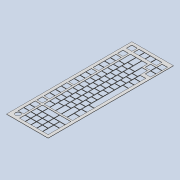
# Autodesk Inventor part: Layout
Saved by Autodesk Inventor 2021 (Build 250183000, 183)
## iProperties
Created: 2021-12-04
Part Number: Layout
Material: Generic
Document SubType Name: Modeling
Designer: Matthew Flooks
Density: 1 g/cm^3
Appearance: Default
Author: Matthew Flooks
Autodesk Inventor part; units mm, degrees
ref_plane "YZ Plane" through (0, 0, 0) normal (1, 0, 0) x (0, 1, 0)
ref_plane "XZ Plane" through (0, 0, 0) normal (0, 1, 0) x (-1, 0, 0)
ref_plane "XY Plane" through (0, 0, 0) normal (0, 0, 1) x (1, 0, 0)
sketch "Sketch1" plane through (0, 0, 0) normal (0, 1, 0) x (-1, 0, 0)
  line L0 (0, 0) -> (19, 0)
  line L1 (19, 0) -> (19, -39.05)
  line L2 (19, -39.05) -> (0, -39.05)
  line L3 (0, -39.05) -> (0, 0)
  line L4 (19, -40.1) -> (0, -40.1)
  line L5 (0, -40.1) -> (0, -59.1)
  line L6 (0, -59.1) -> (19, -59.1)
  line L7 (19, -59.1) -> (19, -40.1)
  line L8 (0, -60.15) -> (39.05, -60.15)
  line L9 (39.05, -60.15) -> (39.05, -79.15)
  line L10 (39.05, -79.15) -> (0, -79.15)
  line L11 (0, -79.15) -> (0, -60.15)
  line L12 (20.05, -59.1) -> (39.05, -59.1)
  line L13 (39.05, -59.1) -> (39.05, -40.1)
  line L14 (39.05, -40.1) -> (20.05, -40.1)
  line L15 (20.05, -40.1) -> (20.05, -59.1)
  line L16 (20.05, -39.05) -> (39.05, -39.05)
  line L17 (39.05, -39.05) -> (39.05, -20.05)
  line L18 (39.05, -20.05) -> (20.05, -20.05)
  line L19 (20.05, -20.05) -> (20.05, -39.05)
  line L20 (20.05, -19) -> (39.05, -19)
  line L21 (39.05, -19) -> (39.05, 0)
  line L22 (39.05, 0) -> (20.05, 0)
  line L23 (20.05, 0) -> (20.05, -19)
  line L24 (40.1, 0) -> (59.1, 0)
  line L25 (59.1, 0) -> (59.1, -19)
  line L26 (59.1, -19) -> (40.1, -19)
  line L27 (40.1, -19) -> (40.1, 0)
  line L28 (40.1, -20.05) -> (59.1, -20.05)
  line L29 (59.1, -20.05) -> (59.1, -39.05)
  line L30 (59.1, -39.05) -> (40.1, -39.05)
  line L31 (40.1, -39.05) -> (40.1, -20.05)
  line L32 (40.1, -40.1) -> (59.1, -40.1)
  line L33 (59.1, -40.1) -> (59.1, -59.1)
  line L34 (59.1, -59.1) -> (40.1, -59.1)
  line L35 (40.1, -59.1) -> (40.1, -40.1)
  line L36 (40.1, -60.15) -> (79.15, -60.15)
  line L37 (79.15, -60.15) -> (79.15, -79.15)
  line L38 (79.15, -79.15) -> (40.1, -79.15)
  line L39 (40.1, -79.15) -> (40.1, -60.15)
  line L40 (60.15, -59.1) -> (79.15, -59.1)
  line L41 (79.15, -59.1) -> (79.15, -40.1)
  line L42 (79.15, -40.1) -> (60.15, -40.1)
  line L43 (60.15, -40.1) -> (60.15, -59.1)
  line L44 (60.15, -39.05) -> (79.15, -39.05)
  line L45 (79.15, -39.05) -> (79.15, -20.05)
  line L46 (79.15, -20.05) -> (60.15, -20.05)
  line L47 (60.15, -20.05) -> (60.15, -39.05)
  line L48 (60.15, -19) -> (79.15, -19)
  line L49 (79.15, -19) -> (79.15, 0)
  line L50 (79.15, 0) -> (60.15, 0)
  line L51 (60.15, 0) -> (60.15, -19)
  line L52 (80.2, 0) -> (99.2, 0)
  line L53 (99.2, 0) -> (99.2, -19)
  line L54 (99.2, -19) -> (80.2, -19)
  line L55 (80.2, -19) -> (80.2, 0)
  line L56 (80.2, -20.05) -> (99.2, -20.05)
  line L57 (99.2, -20.05) -> (99.2, -39.05)
  line L58 (99.2, -39.05) -> (80.2, -39.05)
  line L59 (80.2, -39.05) -> (80.2, -20.05)
  line L60 (80.2, -40.1) -> (99.2, -40.1)
  line L61 (99.2, -40.1) -> (99.2, -59.1)
  line L62 (99.2, -59.1) -> (80.2, -59.1)
  line L63 (80.2, -59.1) -> (80.2, -40.1)
  line L64 (80.2, -60.15) -> (99.2, -60.15)
  line L65 (99.2, -60.15) -> (99.2, -79.15)
  line L66 (99.2, -79.15) -> (80.2, -79.15)
  line L67 (80.2, -79.15) -> (80.2, -60.15)
  line L68 (105.0125, -20.05) -> (124.0125, -20.05)
  line L69 (124.0125, -20.05) -> (124.0125, -39.05)
  line L70 (124.0125, -39.05) -> (105.0125, -39.05)
  line L71 (105.0125, -39.05) -> (105.0125, -20.05)
  line L72 (105.0125, -40.1) -> (124.0125, -40.1)
  line L73 (124.0125, -40.1) -> (124.0125, -59.1)
  line L74 (124.0125, -59.1) -> (105.0125, -59.1)
  line L75 (105.0125, -59.1) -> (105.0125, -40.1)
  line L76 (105.0125, -60.15) -> (124.0125, -60.15)
  line L77 (124.0125, -60.15) -> (124.0125, -79.15)
  line L78 (124.0125, -79.15) -> (105.0125, -79.15)
  line L79 (105.0125, -79.15) -> (105.0125, -60.15)
  line L80 (0, -84.9625) -> (19, -84.9625)
  line L81 (19, -84.9625) -> (19, -108.975)
  line L82 (19, -108.975) -> (0, -108.975)
  line L83 (0, -108.975) -> (0, -84.9625)
  line L84 (0, -110.025) -> (19, -110.025)
  line L85 (19, -110.025) -> (19, -134.0375)
  line L86 (19, -134.0375) -> (0, -134.0375)
  line L87 (0, -134.0375) -> (0, -110.025)
  line L88 (0, -135.0875) -> (19, -135.0875)
  line L89 (19, -135.0875) -> (19, -159.1)
  line L90 (19, -159.1) -> (0, -159.1)
  line L91 (0, -159.1) -> (0, -135.0875)
  line L92 (0, -160.15) -> (19, -160.15)
  line L93 (19, -160.15) -> (19, -278.15)
  line L94 (19, -278.15) -> (0, -278.15)
  line L95 (0, -278.15) -> (0, -160.15)
  line L96 (0, -279.2) -> (19, -279.2)
  line L97 (19, -279.2) -> (19, -298.2)
  line L98 (19, -298.2) -> (0, -298.2)
  line L99 (0, -298.2) -> (0, -279.2)
  line L100 (0, -299.25) -> (19, -299.25)
  line L101 (19, -299.25) -> (19, -318.25)
  line L102 (19, -318.25) -> (0, -318.25)
  line L103 (0, -318.25) -> (0, -299.25)
  line L104 (0, -319.3) -> (19, -319.3)
  line L105 (19, -319.3) -> (19, -338.3)
  line L106 (19, -338.3) -> (0, -338.3)
  line L107 (0, -338.3) -> (0, -319.3)
  line L108 (20.05, -84.9625) -> (39.05, -84.9625)
  line L109 (39.05, -84.9625) -> (39.05, -129.025)
  line L110 (39.05, -129.025) -> (20.05, -129.025)
  line L111 (20.05, -129.025) -> (20.05, -84.9625)
  line L112 (40.1, -84.9625) -> (59.1, -84.9625)
  line L113 (59.1, -84.9625) -> (59.1, -119)
  line L114 (59.1, -119) -> (40.1, -119)
  line L115 (40.1, -119) -> (40.1, -84.9625)
  line L116 (60.15, -84.9625) -> (79.15, -84.9625)
  line L117 (79.15, -84.9625) -> (79.15, -113.9875)
  line L118 (79.15, -113.9875) -> (60.15, -113.9875)
  line L119 (60.15, -113.9875) -> (60.15, -84.9625)
  line L120 (80.2, -84.9625) -> (99.2, -84.9625)
  line L121 (99.2, -84.9625) -> (99.2, -103.9625)
  line L122 (99.2, -103.9625) -> (80.2, -103.9625)
  line L123 (80.2, -103.9625) -> (80.2, -84.9625)
  line L124 (20.05, -130.075) -> (39.05, -130.075)
  line L125 (39.05, -130.075) -> (39.05, -149.075)
  line L126 (39.05, -149.075) -> (20.05, -149.075)
  line L127 (20.05, -149.075) -> (20.05, -130.075)
  line L128 (20.05, -150.125) -> (39.05, -150.125)
  line L129 (39.05, -150.125) -> (39.05, -169.125)
  line L130 (39.05, -169.125) -> (20.05, -169.125)
  line L131 (20.05, -169.125) -> (20.05, -150.125)
  line L132 (20.05, -170.175) -> (39.05, -170.175)
  line L133 (39.05, -170.175) -> (39.05, -189.175)
  line L134 (39.05, -189.175) -> (20.05, -189.175)
  line L135 (20.05, -189.175) -> (20.05, -170.175)
  line L136 (20.05, -190.225) -> (39.05, -190.225)
  line L137 (39.05, -190.225) -> (39.05, -209.225)
  line L138 (39.05, -209.225) -> (20.05, -209.225)
  line L139 (20.05, -209.225) -> (20.05, -190.225)
  line L140 (20.05, -210.275) -> (39.05, -210.275)
  line L141 (39.05, -210.275) -> (39.05, -229.275)
  line L142 (39.05, -229.275) -> (20.05, -229.275)
  line L143 (20.05, -229.275) -> (20.05, -210.275)
  line L144 (20.05, -230.325) -> (39.05, -230.325)
  line L145 (39.05, -230.325) -> (39.05, -249.325)
  line L146 (39.05, -249.325) -> (20.05, -249.325)
  line L147 (20.05, -249.325) -> (20.05, -230.325)
  line L148 (20.05, -250.375) -> (39.05, -250.375)
  line L149 (39.05, -250.375) -> (39.05, -269.375)
  line L150 (39.05, -269.375) -> (20.05, -269.375)
  line L151 (20.05, -269.375) -> (20.05, -250.375)
  line L152 (20.05, -270.425) -> (39.05, -270.425)
  line L153 (39.05, -270.425) -> (39.05, -289.425)
  line L154 (39.05, -289.425) -> (20.05, -289.425)
  line L155 (20.05, -289.425) -> (20.05, -270.425)
  line L156 (20.05, -290.475) -> (39.05, -290.475)
  line L157 (39.05, -290.475) -> (39.05, -309.475)
  line L158 (39.05, -309.475) -> (20.05, -309.475)
  line L159 (20.05, -309.475) -> (20.05, -290.475)
  line L160 (20.05, -329.525) -> (39.05, -329.525)
  line L161 (39.05, -329.525) -> (39.05, -310.525)
  line L162 (39.05, -310.525) -> (20.05, -310.525)
  line L163 (20.05, -310.525) -> (20.05, -329.525)
  line L164 (20.05, -330.575) -> (39.05, -330.575)
  line L165 (39.05, -330.575) -> (39.05, -364.6125)
  line L166 (39.05, -364.6125) -> (20.05, -364.6125)
  line L167 (20.05, -364.6125) -> (20.05, -330.575)
  line L168 (40.1, -120.05) -> (59.1, -120.05)
  line L169 (59.1, -120.05) -> (59.1, -139.05)
  line L170 (59.1, -139.05) -> (40.1, -139.05)
  line L171 (40.1, -139.05) -> (40.1, -120.05)
  line L172 (40.1, -140.1) -> (59.1, -140.1)
  line L173 (59.1, -140.1) -> (59.1, -159.1)
  line L174 (59.1, -159.1) -> (40.1, -159.1)
  line L175 (40.1, -159.1) -> (40.1, -140.1)
  line L176 (40.1, -160.15) -> (59.1, -160.15)
  line L177 (59.1, -160.15) -> (59.1, -179.15)
  line L178 (59.1, -179.15) -> (40.1, -179.15)
  line L179 (40.1, -179.15) -> (40.1, -160.15)
  line L180 (40.1, -180.2) -> (59.1, -180.2)
  line L181 (59.1, -180.2) -> (59.1, -199.2)
  line L182 (59.1, -199.2) -> (40.1, -199.2)
  line L183 (40.1, -199.2) -> (40.1, -180.2)
  line L184 (40.1, -200.25) -> (59.1, -200.25)
  line L185 (59.1, -200.25) -> (59.1, -219.25)
  line L186 (59.1, -219.25) -> (40.1, -219.25)
  line L187 (40.1, -219.25) -> (40.1, -200.25)
  line L188 (59.1, -220.3) -> (40.1, -220.3)
  line L189 (40.1, -220.3) -> (40.1, -239.3)
  line L190 (40.1, -239.3) -> (59.1, -239.3)
  line L191 (59.1, -239.3) -> (59.1, -220.3)
  line L192 (40.1, -240.35) -> (59.1, -240.35)
  line L193 (59.1, -240.35) -> (59.1, -259.35)
  line L194 (59.1, -259.35) -> (40.1, -259.35)
  line L195 (40.1, -259.35) -> (40.1, -240.35)
  line L196 (40.1, -260.4) -> (59.1, -260.4)
  line L197 (59.1, -260.4) -> (59.1, -279.4)
  line L198 (59.1, -279.4) -> (40.1, -279.4)
  line L199 (40.1, -279.4) -> (40.1, -260.4)
  line L200 (40.1, -280.45) -> (59.1, -280.45)
  line L201 (59.1, -280.45) -> (59.1, -299.45)
  line L202 (59.1, -299.45) -> (40.1, -299.45)
  line L203 (40.1, -299.45) -> (40.1, -280.45)
  line L204 (40.1, -300.5) -> (59.1, -300.5)
  line L205 (59.1, -300.5) -> (59.1, -319.5)
  line L206 (59.1, -319.5) -> (40.1, -319.5)
  line L207 (40.1, -319.5) -> (40.1, -300.5)
  line L208 (40.1, -320.55) -> (59.1, -320.55)
  line L209 (59.1, -320.55) -> (59.1, -339.55)
  line L210 (59.1, -339.55) -> (40.1, -339.55)
  line L211 (40.1, -339.55) -> (40.1, -320.55)
  line L212 (40.1, -340.6) -> (59.1, -340.6)
  line L213 (59.1, -340.6) -> (59.1, -384.6625)
  line L214 (59.1, -384.6625) -> (40.1, -384.6625)
  line L215 (40.1, -384.6625) -> (40.1, -340.6)
  line L216 (79.15, -115.0375) -> (60.15, -115.0375)
  line L217 (60.15, -115.0375) -> (60.15, -134.0375)
  line L218 (60.15, -134.0375) -> (79.15, -134.0375)
  line L219 (79.15, -134.0375) -> (79.15, -115.0375)
  line L220 (79.15, -135.0875) -> (60.15, -135.0875)
  line L221 (60.15, -135.0875) -> (60.15, -154.0875)
  line L222 (60.15, -154.0875) -> (79.15, -154.0875)
  line L223 (79.15, -154.0875) -> (79.15, -135.0875)
  line L224 (79.15, -155.1375) -> (60.15, -155.1375)
  line L225 (60.15, -155.1375) -> (60.15, -174.1375)
  line L226 (60.15, -174.1375) -> (79.15, -174.1375)
  line L227 (79.15, -174.1375) -> (79.15, -155.1375)
  line L228 (79.15, -175.1875) -> (60.15, -175.1875)
  line L229 (60.15, -175.1875) -> (60.15, -194.1875)
  line L230 (60.15, -194.1875) -> (79.15, -194.1875)
  line L231 (79.15, -194.1875) -> (79.15, -175.1875)
  line L232 (79.15, -195.2375) -> (60.15, -195.2375)
  line L233 (60.15, -195.2375) -> (60.15, -214.2375)
  line L234 (60.15, -214.2375) -> (79.15, -214.2375)
  line L235 (79.15, -214.2375) -> (79.15, -195.2375)
  line L236 (79.15, -215.2875) -> (60.15, -215.2875)
  line L237 (60.15, -215.2875) -> (60.15, -234.2875)
  line L238 (60.15, -234.2875) -> (79.15, -234.2875)
  line L239 (79.15, -234.2875) -> (79.15, -215.2875)
  line L240 (79.15, -235.3375) -> (60.15, -235.3375)
  line L241 (60.15, -235.3375) -> (60.15, -254.3375)
  line L242 (60.15, -254.3375) -> (79.15, -254.3375)
  line L243 (79.15, -254.3375) -> (79.15, -235.3375)
  line L244 (79.15, -255.3875) -> (60.15, -255.3875)
  line L245 (60.15, -255.3875) -> (60.15, -274.3875)
  line L246 (60.15, -274.3875) -> (79.15, -274.3875)
  line L247 (79.15, -274.3875) -> (79.15, -255.3875)
  line L248 (79.15, -275.4375) -> (60.15, -275.4375)
  line L249 (60.15, -275.4375) -> (60.15, -294.4375)
  line L250 (60.15, -294.4375) -> (79.15, -294.4375)
  line L251 (79.15, -294.4375) -> (79.15, -275.4375)
  line L252 (79.15, -295.4875) -> (60.15, -295.4875)
  line L253 (60.15, -295.4875) -> (60.15, -314.4875)
  line L254 (60.15, -314.4875) -> (79.15, -314.4875)
  line L255 (79.15, -314.4875) -> (79.15, -295.4875)
  line L256 (60.15, -315.5375) -> (79.15, -315.5375)
  line L257 (79.15, -315.5375) -> (79.15, -334.5375)
  line L258 (79.15, -334.5375) -> (60.15, -334.5375)
  line L259 (60.15, -334.5375) -> (60.15, -315.5375)
  line L260 (60.15, -335.5875) -> (79.15, -335.5875)
  line L261 (79.15, -335.5875) -> (79.15, -354.5875)
  line L262 (79.15, -354.5875) -> (60.15, -354.5875)
  line L263 (60.15, -354.5875) -> (60.15, -335.5875)
  line L264 (79.15, -355.6375) -> (60.15, -355.6375)
  line L265 (60.15, -355.6375) -> (60.15, -384.6625)
  line L266 (60.15, -384.6625) -> (79.15, -384.6625)
  line L267 (79.15, -384.6625) -> (79.15, -355.6375)
  line L268 (80.2, -105.0125) -> (99.2, -105.0125)
  line L269 (99.2, -105.0125) -> (99.2, -124.0125)
  line L270 (99.2, -124.0125) -> (80.2, -124.0125)
  line L271 (80.2, -124.0125) -> (80.2, -105.0125)
  line L272 (80.2, -125.0625) -> (99.2, -125.0625)
  line L273 (99.2, -125.0625) -> (99.2, -144.0625)
  line L274 (99.2, -144.0625) -> (80.2, -144.0625)
  line L275 (80.2, -144.0625) -> (80.2, -125.0625)
  line L276 (80.2, -145.1125) -> (99.2, -145.1125)
  line L277 (99.2, -145.1125) -> (99.2, -164.1125)
  line L278 (99.2, -164.1125) -> (80.2, -164.1125)
  line L279 (80.2, -164.1125) -> (80.2, -145.1125)
  line L280 (80.2, -165.1625) -> (99.2, -165.1625)
  line L281 (99.2, -165.1625) -> (99.2, -184.1625)
  line L282 (99.2, -184.1625) -> (80.2, -184.1625)
  line L283 (80.2, -184.1625) -> (80.2, -165.1625)
  line L284 (80.2, -185.2125) -> (99.2, -185.2125)
  line L285 (99.2, -185.2125) -> (99.2, -204.2125)
  line L286 (99.2, -204.2125) -> (80.2, -204.2125)
  line L287 (80.2, -204.2125) -> (80.2, -185.2125)
  line L288 (80.2, -205.2625) -> (99.2, -205.2625)
  line L289 (99.2, -205.2625) -> (99.2, -224.2625)
  line L290 (99.2, -224.2625) -> (80.2, -224.2625)
  line L291 (80.2, -224.2625) -> (80.2, -205.2625)
  line L292 (80.2, -225.3125) -> (99.2, -225.3125)
  line L293 (99.2, -225.3125) -> (99.2, -244.3125)
  line L294 (99.2, -244.3125) -> (80.2, -244.3125)
  line L295 (80.2, -244.3125) -> (80.2, -225.3125)
  line L296 (80.2, -245.3625) -> (99.2, -245.3625)
  line L297 (99.2, -245.3625) -> (99.2, -264.3625)
  line L298 (99.2, -264.3625) -> (80.2, -264.3625)
  line L299 (80.2, -264.3625) -> (80.2, -245.3625)
  line L300 (80.2, -265.4125) -> (99.2, -265.4125)
  line L301 (99.2, -265.4125) -> (99.2, -284.4125)
  line L302 (99.2, -284.4125) -> (80.2, -284.4125)
  line L303 (80.2, -284.4125) -> (80.2, -265.4125)
  line L304 (80.2, -285.4625) -> (99.2, -285.4625)
  line L305 (99.2, -285.4625) -> (99.2, -304.4625)
  line L306 (99.2, -304.4625) -> (80.2, -304.4625)
  line L307 (80.2, -304.4625) -> (80.2, -285.4625)
  line L308 (80.2, -305.5125) -> (99.2, -305.5125)
  line L309 (99.2, -305.5125) -> (99.2, -324.5125)
  line L310 (99.2, -324.5125) -> (80.2, -324.5125)
  line L311 (80.2, -324.5125) -> (80.2, -305.5125)
  line L312 (80.2, -325.5625) -> (99.2, -325.5625)
  line L313 (99.2, -325.5625) -> (99.2, -344.5625)
  line L314 (99.2, -344.5625) -> (80.2, -344.5625)
  line L315 (80.2, -344.5625) -> (80.2, -325.5625)
  line L316 (80.2, -345.6125) -> (99.2, -345.6125)
  line L317 (99.2, -345.6125) -> (99.2, -384.6625)
  line L318 (99.2, -384.6625) -> (80.2, -384.6625)
  line L319 (80.2, -384.6625) -> (80.2, -345.6125)
  line L320 (105.0125, -84.9625) -> (124.0125, -84.9625)
  line L321 (124.0125, -84.9625) -> (124.0125, -103.9625)
  line L322 (124.0125, -103.9625) -> (105.0125, -103.9625)
  line L323 (105.0125, -103.9625) -> (105.0125, -84.9625)
  line L324 (124.0125, -109.775) -> (105.0125, -109.775)
  line L325 (105.0125, -109.775) -> (105.0125, -128.775)
  line L326 (105.0125, -128.775) -> (124.0125, -128.775)
  line L327 (124.0125, -128.775) -> (124.0125, -109.775)
  line L328 (124.0125, -129.825) -> (105.0125, -129.825)
  line L329 (105.0125, -129.825) -> (105.0125, -148.825)
  line L330 (105.0125, -148.825) -> (124.0125, -148.825)
  line L331 (124.0125, -148.825) -> (124.0125, -129.825)
  line L332 (124.0125, -149.875) -> (105.0125, -149.875)
  line L333 (105.0125, -149.875) -> (105.0125, -168.875)
  line L334 (105.0125, -168.875) -> (124.0125, -168.875)
  line L335 (124.0125, -168.875) -> (124.0125, -149.875)
  line L336 (124.0125, -169.925) -> (105.0125, -169.925)
  line L337 (105.0125, -169.925) -> (105.0125, -188.925)
  line L338 (105.0125, -188.925) -> (124.0125, -188.925)
  line L339 (124.0125, -188.925) -> (124.0125, -169.925)
  line L340 (124.0125, -213.7375) -> (105.0125, -213.7375)
  line L341 (105.0125, -213.7375) -> (105.0125, -194.7375)
  line L342 (105.0125, -194.7375) -> (124.0125, -194.7375)
  line L343 (124.0125, -194.7375) -> (124.0125, -213.7375)
  line L344 (124.0125, -214.7875) -> (105.0125, -214.7875)
  line L345 (105.0125, -214.7875) -> (105.0125, -233.7875)
  line L346 (105.0125, -233.7875) -> (124.0125, -233.7875)
  line L347 (124.0125, -233.7875) -> (124.0125, -214.7875)
  line L348 (124.0125, -234.8375) -> (105.0125, -234.8375)
  line L349 (105.0125, -234.8375) -> (105.0125, -253.8375)
  line L350 (105.0125, -253.8375) -> (124.0125, -253.8375)
  line L351 (124.0125, -253.8375) -> (124.0125, -234.8375)
  line L352 (124.0125, -254.8875) -> (105.0125, -254.8875)
  line L353 (105.0125, -254.8875) -> (105.0125, -273.8875)
  line L354 (105.0125, -273.8875) -> (124.0125, -273.8875)
  line L355 (124.0125, -273.8875) -> (124.0125, -254.8875)
  line L356 (124.0125, -279.7) -> (105.0125, -279.7)
  line L357 (105.0125, -279.7) -> (105.0125, -298.7)
  line L358 (105.0125, -298.7) -> (124.0125, -298.7)
  line L359 (124.0125, -298.7) -> (124.0125, -279.7)
  line L360 (124.0125, -299.75) -> (105.0125, -299.75)
  line L361 (105.0125, -299.75) -> (105.0125, -318.75)
  line L362 (105.0125, -318.75) -> (124.0125, -318.75)
  line L363 (124.0125, -318.75) -> (124.0125, -299.75)
  line L364 (124.0125, -319.8) -> (105.0125, -319.8)
  line L365 (105.0125, -319.8) -> (105.0125, -338.8)
  line L366 (105.0125, -338.8) -> (124.0125, -338.8)
  line L367 (124.0125, -338.8) -> (124.0125, -319.8)
  line L368 (124.0125, -339.85) -> (105.0125, -339.85)
  line L369 (105.0125, -339.85) -> (105.0125, -358.85)
  line L370 (105.0125, -358.85) -> (124.0125, -358.85)
  line L371 (124.0125, -358.85) -> (124.0125, -339.85)
  line L372 (124.0125, -364.6625) -> (105.0125, -364.6625)
  line L373 (105.0125, -364.6625) -> (105.0125, -383.6625)
  line L374 (105.0125, -383.6625) -> (124.0125, -383.6625)
  line L375 (124.0125, -383.6625) -> (124.0125, -364.6625)
  line L376 (124.0125, -395.2375) -> (105.0125, -395.2375)
  line L377 (105.0125, -395.2375) -> (105.0125, -414.2375)
  line L378 (105.0125, -414.2375) -> (124.0125, -414.2375)
  line L379 (124.0125, -414.2375) -> (124.0125, -395.2375)
  line L380 (14.2375, -350.375) -> (-4.7625, -350.375)
  line L381 (-4.7625, -350.375) -> (-4.7625, -369.375)
  line L382 (-4.7625, -369.375) -> (14.2375, -369.375)
  line L383 (14.2375, -369.375) -> (14.2375, -350.375)
  line L384 (14.2375, -370.425) -> (-4.7625, -370.425)
  line L385 (-4.7625, -370.425) -> (-4.7625, -389.425)
  line L386 (-4.7625, -389.425) -> (14.2375, -389.425)
  line L387 (14.2375, -389.425) -> (14.2375, -370.425)
  line L388 (14.2375, -390.475) -> (-4.7625, -390.475)
  line L389 (-4.7625, -390.475) -> (-4.7625, -409.475)
  line L390 (-4.7625, -409.475) -> (14.2375, -409.475)
  line L391 (14.2375, -409.475) -> (14.2375, -390.475)
  line L392 (15.2875, -389.425) -> (34.2875, -389.425)
  line L393 (34.2875, -389.425) -> (34.2875, -370.425)
  line L394 (34.2875, -370.425) -> (15.2875, -370.425)
  line L395 (15.2875, -370.425) -> (15.2875, -389.425)
  line L396 (20.05, -395.2375) -> (39.05, -395.2375)
  line L397 (39.05, -395.2375) -> (39.05, -414.2375)
  line L398 (39.05, -414.2375) -> (20.05, -414.2375)
  line L399 (20.05, -414.2375) -> (20.05, -395.2375)
  line L400 (60.15, -395.2375) -> (79.15, -395.2375)
  line L401 (79.15, -395.2375) -> (79.15, -414.2375)
  line L402 (79.15, -414.2375) -> (60.15, -414.2375)
  line L403 (60.15, -414.2375) -> (60.15, -395.2375)
  line L404 (80.2, -395.2375) -> (99.2, -395.2375)
  line L405 (99.2, -395.2375) -> (99.2, -414.2375)
  line L406 (99.2, -414.2375) -> (80.2, -414.2375)
  line L407 (80.2, -414.2375) -> (80.2, -395.2375)
  line L408 (59.1, -395.2375) -> (40.1, -395.2375)
  line L409 (40.1, -395.2375) -> (40.1, -414.2375)
  line L410 (40.1, -414.2375) -> (59.1, -414.2375)
  line L411 (59.1, -414.2375) -> (59.1, -395.2375)
  circle A0 centre (114.5125, -10) radius 8.525
  line L412 (-10, 10) -> (134.0125, 10)
  line L413 (134.0125, 10) -> (134.0125, -424.2375)
  line L414 (134.0125, -424.2375) -> (-10, -424.2375)
  line L415 (-10, -424.2375) -> (-10, 10)
  line L416 (114.5125, -20.05) -> (114.5125, -10) construction
  point P0 (0, 0)
  dimension "d0" = 39.05
  dimension "d1" = 19
  dimension "d2" = 0
  dimension "d3" = 0
  dimension "d4" = 19
  dimension "d5" = 1.05
  dimension "d6" = 39.05
  dimension "d7" = 19
  dimension "d8" = 1.05
  dimension "d10" = 19
  dimension "d12" = 19
  dimension "d13" = 19
  dimension "d15" = 19
  dimension "d16" = 19
  dimension "d17" = 1.05
  dimension "d18" = 1.05
  dimension "d21" = 19
  dimension "d25" = 1.05
  dimension "d26" = 39.05
  dimension "d27" = 19
  dimension "d33" = 1.05
  dimension "d34" = 19
  dimension "d37" = 24.0125
  dimension "d38" = 5.8125
  dimension "d39" = 24.0125
  dimension "d40" = 24.0125
  dimension "d41" = 1.05
  dimension "d42" = 1.05
  dimension "d43" = 1.05
  dimension "d44" = 1.05
  dimension "d45" = 1.05
  dimension "d46" = 1.05
  dimension "d47" = 19
  dimension "d48" = 19
  dimension "d49" = 19
  dimension "d50" = 118
  dimension "d51" = 44.0625
  dimension "d52" = 1.05
  dimension "d53" = 34.0375
  dimension "d54" = 29.025
  dimension "d55" = 19
  dimension "d56" = 1.05
  dimension "d57" = 1.05
  dimension "d58" = 1.05
  dimension "d59" = 1.05
  dimension "d60" = 1.05
  dimension "d61" = 1.05
  dimension "d62" = 1.05
  dimension "d63" = 1.05
  dimension "d64" = 1.05
  dimension "d66" = 19
  dimension "d67" = 19
  dimension "d68" = 19
  dimension "d69" = 19
  dimension "d70" = 19
  dimension "d71" = 19
  dimension "d72" = 19
  dimension "d73" = 19
  dimension "d74" = 19
  dimension "d75" = 19
  dimension "d76" = 1.05
  dimension "d77" = 1.05
  dimension "d78" = 34.0375
  dimension "d79" = 19
  constraints: 834 end point, 208 parallel, 139 point on line, 104 horizontal, 104 perpendicular, 76 collinear, 1 centre point, 1 midpoint, 1 vertical
  measures "d0" distance of L2.end L0.start
  measures "d1" distance of L1.end L2.end
  measures "d2" distance from line of point (0, 0) L0
  measures "d3" distance from line of point (0, 0) L3
  measures "d4" distance of L4.end L5.end
  measures "d5" distance between parallel lines of L2 L4
  measures "d6" distance of L9.end L10.end
  measures "d7" distance of L10.end L8.start
  measures "d8" distance between parallel lines of L6 L8
  measures "d10" distance of L12.end L13.end
  measures "d12" distance of L17.end L18.end
  measures "d13" distance of L16.end L17.end
  measures "d15" distance of L20.end L21.end
  measures "d16" distance of L21.end L22.end
  measures "d17" distance between parallel lines of L1 L23
  measures "d18" distance between parallel lines of L18 L20
  measures "d21" distance of L24.start L24.end
  measures "d25" distance between parallel lines of L21 L27
  measures "d26" distance of L37.end L38.end
  measures "d27" distance of L41.end L42.end
  measures "d33" distance between parallel lines of L41 L63
  measures "d34" distance of L52.start L52.end
  measures "d37" distance of L82.end L80.start
  measures "d38" distance between parallel lines of L10 L80
  measures "d39" distance of L86.end L84.start
  measures "d40" distance of L90.end L88.start
  measures "d41" distance between parallel lines of L82 L84
  measures "d42" distance between parallel lines of L88 L86
  measures "d43" distance between parallel lines of L92 L90
  measures "d44" distance between parallel lines of L96 L94
  measures "d45" distance between parallel lines of L100 L98
  measures "d46" distance between parallel lines of L104 L102
  measures "d47" distance of L98.end L96.start
  measures "d48" distance of L102.end L100.start
  measures "d49" distance of L106.end L104.start
  measures "d50" distance of L94.end L92.start
  measures "d51" distance of L110.end L108.start
  measures "d52" distance between parallel lines of L111 L81
  measures "d53" distance of L114.end L112.start
  measures "d54" distance of L118.end L116.start
  measures "d55" distance of L122.end L120.start
  measures "d56" distance between parallel lines of L124 L110
  measures "d57" distance between parallel lines of L128 L126
  measures "d58" distance between parallel lines of L132 L130
  measures "d59" distance between parallel lines of L136 L134
  measures "d60" distance between parallel lines of L140 L138
  measures "d61" distance between parallel lines of L144 L142
  measures "d62" distance between parallel lines of L148 L146
  measures "d63" distance between parallel lines of L152 L150
  measures "d64" distance between parallel lines of L156 L154
  measures "d66" distance of L126.end L124.start
  measures "d67" distance of L130.end L128.start
  measures "d68" distance of L134.end L132.start
  measures "d69" distance of L138.end L136.start
  measures "d70" distance of L142.end L140.start
  measures "d71" distance of L146.end L144.start
  measures "d72" distance of L150.end L148.start
  measures "d73" distance of L154.end L152.start
  measures "d74" distance of L158.end L156.start
  measures "d75" distance of L162.end L160.start
  measures "d76" distance between parallel lines of L158 L162
  measures "d77" distance between parallel lines of L160 L164
  measures "d78" distance of L166.end L164.start
  measures "d79" distance of L168.end L169.end
extrude "Extrusion2" add sketch "Sketch1" along normal blind 1
equation "\"d0\" = u2"
equation "\"d1\" = u1"
equation "\"d4\" = u1"
equation "\"d5\" = spacing"
equation "\"d6\" = u2"
equation "\"d7\" = u1"
equation "\"d8\" = spacing"
equation "\"d10\" = u1"
equation "\"d12\" = u1"
equation "\"d13\" = u1"
equation "\"d15\" = u1"
equation "\"d16\" = u1"
equation "\"d17\" = spacing"
equation "\"d18\" = spacing"
equation "\"d21\" = u1"
equation "\"d25\" = spacing"
equation "\"d26\" = u2"
equation "\"d27\" = u1"
equation "\"d33\" = spacing"
equation "\"d34\" = u1"
equation "\"d37\" = u125"
equation "\"d39\" = u125"
equation "\"d40\" = u125"
equation "\"d41\" = spacing"
equation "\"d42\" = spacing"
equation "\"d43\" = spacing"
equation "\"d44\" = spacing"
equation "\"d45\" = spacing"
equation "\"d46\" = spacing"
equation "\"d47\" = u1"
equation "\"d48\" = u1"
equation "\"d49\" = u1"
equation "\"d50\" = uspace"
equation "\"d51\" = u225"
equation "\"d52\" = spacing"
equation "\"d53\" = u175"
equation "\"d54\" = u15"
equation "\"d55\" = u1"
equation "\"d56\" = spacing"
equation "\"d57\" = spacing"
equation "\"d58\" = spacing"
equation "\"d59\" = spacing"
equation "\"d60\" = spacing"
equation "\"d61\" = spacing"
equation "\"d62\" = spacing"
equation "\"d63\" = spacing"
equation "\"d64\" = spacing"
equation "\"d66\" = u1"
equation "\"d67\" = u1"
equation "\"d68\" = u1"
equation "\"d69\" = u1"
equation "\"d70\" = u1"
equation "\"d71\" = u1"
equation "\"d72\" = u1"
equation "\"d73\" = u1"
equation "\"d74\" = u1"
equation "\"d75\" = u1"
equation "\"d76\" = spacing"
equation "\"d77\" = spacing"
equation "\"d78\" = u175"
equation "\"d79\" = u1"
equation "\"u2\" = 39.05"
equation "\"u1\" = 19"
equation "\"u125\" = 24.0125"
equation "\"u15\" = 29.025"
equation "\"u175\" = 34.0375"
equation "\"u225\" = 44.0625"
equation "\"u25\" = 49.075"
equation "\"u275\" = 54.0875"
equation "\"spacing\" = 1.05"
equation "\"uspace\" = 118"
equation "\"spacing2\" = 5.8125"
equation "\"size\" = 20.05"
body "Solid2"
